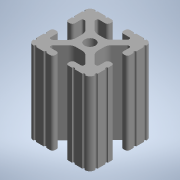
# Autodesk Inventor part: Extrusion 15 x 15 x 2
Saved by Autodesk Inventor 2022.2 (Build 262287010, 287A)
## iProperties
Category: PARTsolutions
Company: 8020
Part Number: Extrusion 15 x 15 x 2
Material: Generic
Catalog Web Link: www.cadenas.de
Description: 1515, 1515-Black, 1515-Black-FB-T-Slotted Profile - 15 Series
Vendor: 8020
Document SubType Name: Modeling
Designer: partserver
Manufacturer: 8020
Mass: 37.8035 g
Surface Area: 185.379 cm^2
Volume: 37.8035 cm^3
Density: 1 g/cm^3
Appearance: PSOLRGB-191-191-191
PSOL_IDENT_0: {$CADENAS_DATA\23d-libs\8020\inch\profiles\15_series\1515.prj},192 {VTYP=3D},{NB=1515-2-CL},{LINA=15
PSOL_IDENT_1: 15-2},{NN=1515, 1515-Black, 1515-Black-FB},{DATE=31.07.2020 09:21:23},{GEOMDATE=09.02.2018 15:39:16}
PSOL_IDENT_2: ,{VERSION=},{LINEID=10},{WBVAR=FINISH,LS,L},{WBNUMERIC=L}  {NB=1515-2-CL},{LINA=1515-2},{KT=DUMMY},{
PSOL_IDENT_3: PN=1515-2},{SERIES=1515},{MAT=6105-T5 Aluminum},{FINISH=CA},{W=1.3433},{LS=-CL},{L=2.000},{LALG=[1:2
PSOL_IDENT_4: 42/0.005]},{LPN= },{CLR=.75,.75,.75}
NB: 1515-2-CL
NN: 1515, 1515-Black, 1515-Black-FB
NT: T-Slotted Profile - 15 Series
NBSYN: $PN.$LS.
LINA: 1515-2
CATALOG: 80/20
PN: 1515-2
SERIES: 1515
MAT: 6105-T5 Aluminum
FINISH: Clear Anodize
W: 1.3433
LS: Custom Length
L: 2
SUPPLIER: 8020
ARTICLENO: 1515-2-CL
BOMINFO: 1515-2
CREATOR: CADENAS GmbH
Title: 1515-2
Author: Cadenas PARTsolutions
Comments: T-Slotted Profile - 15 Series
Autodesk Inventor part; units mm, degrees
ref_plane "YZ Plane" through (0, 0, 0) normal (1, 0, 0) x (0, 1, 0)
ref_plane "XZ Plane" through (0, 0, 0) normal (0, 1, 0) x (-1, 0, 0)
ref_plane "XY Plane" through (0, 0, 0) normal (0, 0, 1) x (1, 0, 0)
sketch "Sketch_1" plane through (0, 0, 0) normal (0, 0, 1) x (1, 0, 0)
  arc A0 (-15.8475, 19.05) -> (-19.05, 15.8475) centre (-15.8751, 15.8751) ccw
  arc A1 (-19.05, 14.3277) -> (-19.05, 15.8475) centre (-18.9933, 15.0876) ccw
  line L0 (-19.05, 14.3277) -> (-19.05, 9.4961)
  arc A2 (-19.05, 7.9763) -> (-19.05, 9.4961) centre (-18.9933, 8.7362) ccw
  line L1 (-19.05, 7.9763) -> (-19.05, 5.6176)
  arc A3 (-19.05, 5.6176) -> (-17.4964, 4.064) centre (-17.4964, 5.6176) ccw
  line L2 (-17.4964, 4.064) -> (-16.5396, 4.064)
  arc A4 (-16.5396, 4.064) -> (-14.986, 5.6176) centre (-16.5396, 5.6176) ccw
  line L3 (-14.986, 5.6176) -> (-14.986, 9.3853)
  arc A5 (-14.0843, 10.287) -> (-14.986, 9.3853) centre (-14.0843, 9.3853) ccw
  line L4 (-14.0843, 10.287) -> (-13.516, 10.287)
  arc A6 (-12.8784, 10.0229) -> (-13.516, 10.287) centre (-13.516, 9.3853) ccw
  line L5 (-12.8784, 10.0229) -> (-8.1476, 5.2921)
  arc A7 (-6.7564, 1.9335) -> (-8.1476, 5.2921) centre (-11.5062, 1.9335) ccw
  line L6 (-6.7564, 1.9335) -> (-6.7564, -1.9335)
  arc A8 (-8.1476, -5.2921) -> (-6.7564, -1.9335) centre (-11.5062, -1.9335) ccw
  line L7 (-8.1476, -5.2921) -> (-12.8784, -10.0229)
  arc A9 (-13.516, -10.287) -> (-12.8784, -10.0229) centre (-13.516, -9.3853) ccw
  line L8 (-13.516, -10.287) -> (-14.0843, -10.287)
  arc A10 (-14.986, -9.3853) -> (-14.0843, -10.287) centre (-14.0843, -9.3853) ccw
  line L9 (-14.986, -9.3853) -> (-14.986, -5.6176)
  arc A11 (-14.986, -5.6176) -> (-16.5396, -4.064) centre (-16.5396, -5.6176) ccw
  line L10 (-16.5396, -4.064) -> (-17.4964, -4.064)
  arc A12 (-17.4964, -4.064) -> (-19.05, -5.6176) centre (-17.4964, -5.6176) ccw
  line L11 (-19.05, -5.6176) -> (-19.05, -7.9763)
  arc A13 (-19.05, -9.4961) -> (-19.05, -7.9763) centre (-18.9933, -8.7362) ccw
  line L12 (-19.05, -9.4961) -> (-19.05, -14.3277)
  arc A14 (-19.05, -15.8475) -> (-19.05, -14.3277) centre (-18.9933, -15.0876) ccw
  arc A15 (-19.05, -15.8475) -> (-15.8475, -19.05) centre (-15.8751, -15.8751) ccw
  arc A16 (-14.3277, -19.05) -> (-15.8475, -19.05) centre (-15.0876, -18.9933) ccw
  line L13 (-14.3277, -19.05) -> (-9.4961, -19.05)
  arc A17 (-7.9763, -19.05) -> (-9.4961, -19.05) centre (-8.7362, -18.9933) ccw
  line L14 (-7.9763, -19.05) -> (-5.6176, -19.05)
  arc A18 (-5.6176, -19.05) -> (-4.064, -17.4964) centre (-5.6176, -17.4964) ccw
  line L15 (-4.064, -17.4964) -> (-4.064, -16.5396)
  arc A19 (-4.064, -16.5396) -> (-5.6176, -14.986) centre (-5.6176, -16.5396) ccw
  line L16 (-5.6176, -14.986) -> (-9.3853, -14.986)
  arc A20 (-10.287, -14.0843) -> (-9.3853, -14.986) centre (-9.3853, -14.0843) ccw
  line L17 (-10.287, -14.0843) -> (-10.287, -13.5524)
  arc A21 (-10.0229, -12.9148) -> (-10.287, -13.5524) centre (-9.3853, -13.5524) ccw
  line L18 (-10.0229, -12.9148) -> (-5.2522, -8.144)
  arc A22 (-1.9022, -6.7564) -> (-5.2522, -8.144) centre (-1.9022, -11.494) ccw
  line L19 (-1.9022, -6.7564) -> (1.9022, -6.7564)
  arc A23 (5.2522, -8.144) -> (1.9022, -6.7564) centre (1.9022, -11.494) ccw
  line L20 (5.2522, -8.144) -> (10.0229, -12.9148)
  arc A24 (10.287, -13.5524) -> (10.0229, -12.9148) centre (9.3853, -13.5524) ccw
  line L21 (10.287, -13.5524) -> (10.287, -14.0843)
  arc A25 (9.3853, -14.986) -> (10.287, -14.0843) centre (9.3853, -14.0843) ccw
  line L22 (9.3853, -14.986) -> (5.6176, -14.986)
  arc A26 (5.6176, -14.986) -> (4.064, -16.5396) centre (5.6176, -16.5396) ccw
  line L23 (4.064, -16.5396) -> (4.064, -17.4964)
  arc A27 (4.064, -17.4964) -> (5.6176, -19.05) centre (5.6176, -17.4964) ccw
  line L24 (5.6176, -19.05) -> (7.9763, -19.05)
  arc A28 (9.4961, -19.05) -> (7.9763, -19.05) centre (8.7362, -18.9933) ccw
  line L25 (9.4961, -19.05) -> (14.3277, -19.05)
  arc A29 (15.8475, -19.05) -> (14.3277, -19.05) centre (15.0876, -18.9933) ccw
  arc A30 (15.8475, -19.05) -> (19.05, -15.8475) centre (15.8751, -15.8751) ccw
  arc A31 (19.05, -14.3277) -> (19.05, -15.8475) centre (18.9933, -15.0876) ccw
  line L26 (19.05, -14.3277) -> (19.05, -9.4961)
  arc A32 (19.05, -7.9763) -> (19.05, -9.4961) centre (18.9933, -8.7362) ccw
  line L27 (19.05, -7.9763) -> (19.05, -5.6176)
  arc A33 (19.05, -5.6176) -> (17.4964, -4.064) centre (17.4964, -5.6176) ccw
  line L28 (17.4964, -4.064) -> (16.5396, -4.064)
  arc A34 (16.5396, -4.064) -> (14.986, -5.6176) centre (16.5396, -5.6176) ccw
  line L29 (14.986, -5.6176) -> (14.986, -9.3853)
  arc A35 (14.0843, -10.287) -> (14.986, -9.3853) centre (14.0843, -9.3853) ccw
  line L30 (14.0843, -10.287) -> (13.516, -10.287)
  arc A36 (12.8784, -10.0229) -> (13.516, -10.287) centre (13.516, -9.3853) ccw
  line L31 (12.8784, -10.0229) -> (8.1476, -5.2921)
  arc A37 (6.7564, -1.9335) -> (8.1476, -5.2921) centre (11.5062, -1.9335) ccw
  line L32 (6.7564, -1.9335) -> (6.7564, 1.9335)
  arc A38 (8.1476, 5.2921) -> (6.7564, 1.9335) centre (11.5062, 1.9335) ccw
  line L33 (8.1476, 5.2921) -> (12.8784, 10.0229)
  arc A39 (13.516, 10.287) -> (12.8784, 10.0229) centre (13.516, 9.3853) ccw
  line L34 (13.516, 10.287) -> (14.0843, 10.287)
  arc A40 (14.986, 9.3853) -> (14.0843, 10.287) centre (14.0843, 9.3853) ccw
  line L35 (14.986, 9.3853) -> (14.986, 5.6176)
  arc A41 (14.986, 5.6176) -> (16.5396, 4.064) centre (16.5396, 5.6176) ccw
  line L36 (16.5396, 4.064) -> (17.4964, 4.064)
  arc A42 (17.4964, 4.064) -> (19.05, 5.6176) centre (17.4964, 5.6176) ccw
  line L37 (19.05, 5.6176) -> (19.05, 7.9763)
  arc A43 (19.05, 9.4961) -> (19.05, 7.9763) centre (18.9933, 8.7362) ccw
  line L38 (19.05, 9.4961) -> (19.05, 14.3277)
  arc A44 (19.05, 15.8475) -> (19.05, 14.3277) centre (18.9933, 15.0876) ccw
  arc A45 (19.05, 15.8475) -> (15.8475, 19.05) centre (15.8751, 15.8751) ccw
  arc A46 (14.3277, 19.05) -> (15.8475, 19.05) centre (15.0876, 18.9933) ccw
  line L39 (14.3277, 19.05) -> (9.4982, 19.05)
  arc A47 (7.9742, 19.05) -> (9.4982, 19.05) centre (8.7362, 19.05) ccw
  line L40 (7.9742, 19.05) -> (5.6176, 19.05)
  arc A48 (5.6176, 19.05) -> (4.064, 17.4964) centre (5.6176, 17.4964) ccw
  line L41 (4.064, 17.4964) -> (4.064, 16.5396)
  arc A49 (4.064, 16.5396) -> (5.6176, 14.986) centre (5.6176, 16.5396) ccw
  line L42 (5.6176, 14.986) -> (9.3853, 14.986)
  arc A50 (10.287, 14.0843) -> (9.3853, 14.986) centre (9.3853, 14.0843) ccw
  line L43 (10.287, 14.0843) -> (10.287, 13.5524)
  arc A51 (10.0229, 12.9148) -> (10.287, 13.5524) centre (9.3853, 13.5524) ccw
  line L44 (10.0229, 12.9148) -> (5.2522, 8.144)
  arc A52 (1.9022, 6.7564) -> (5.2522, 8.144) centre (1.9022, 11.494) ccw
  line L45 (1.9022, 6.7564) -> (-1.9022, 6.7564)
  arc A53 (-5.2522, 8.144) -> (-1.9022, 6.7564) centre (-1.9022, 11.494) ccw
  line L46 (-5.2522, 8.144) -> (-10.0229, 12.9148)
  arc A54 (-10.287, 13.5524) -> (-10.0229, 12.9148) centre (-9.3853, 13.5524) ccw
  line L47 (-10.287, 13.5524) -> (-10.287, 14.0843)
  arc A55 (-9.3853, 14.986) -> (-10.287, 14.0843) centre (-9.3853, 14.0843) ccw
  line L48 (-9.3853, 14.986) -> (-5.6176, 14.986)
  arc A56 (-5.6176, 14.986) -> (-4.064, 16.5396) centre (-5.6176, 16.5396) ccw
  line L49 (-4.064, 16.5396) -> (-4.064, 17.4964)
  arc A57 (-4.064, 17.4964) -> (-5.6176, 19.05) centre (-5.6176, 17.4964) ccw
  line L50 (-5.6176, 19.05) -> (-7.9742, 19.05)
  arc A58 (-9.4982, 19.05) -> (-7.9742, 19.05) centre (-8.7362, 19.05) ccw
  line L51 (-9.4982, 19.05) -> (-14.3277, 19.05)
  arc A59 (-15.8475, 19.05) -> (-14.3277, 19.05) centre (-15.0876, 18.9933) ccw
  circle A60 centre (0, 0) radius 3.3274
  constraints: 120 point on circle, 104 end point, 61 centre point
extrude "Extrusion1" add sketch "Sketch_1" against normal blind 50.8
ref_plane "b1_XY" through (-19.05, 0, -25.4) normal (1, 0, 0) x (0, 0, -1)
ref_plane "b1_YZ" through (-19.05, 0, -25.4) normal (0, 0, -1) x (0, 1, 0)
ref_plane "b1_ZX" through (-19.05, 0, -25.4) normal (0, 1, 0) x (1, 0, 0)
ref_plane "b2_XY" through (19.05, 0, -25.4) normal (1, 0, 0) x (0, 0, -1)
ref_plane "b2_YZ" through (19.05, 0, -25.4) normal (0, 0, -1) x (0, 1, 0)
ref_plane "b2_ZX" through (19.05, 0, -25.4) normal (0, 1, 0) x (1, 0, 0)
ref_plane "profile1515_XY" through (0, 0, -25.4) normal (0, 0, 1) x (1, 0, 0)
ref_plane "profile1515_YZ" through (0, 0, -25.4) normal (1, 0, 0) x (0, 1, 0)
ref_plane "profile1515_ZX" through (0, 0, -25.4) normal (0, 1, 0) x (0, 0, 1)
body "Solid1"
